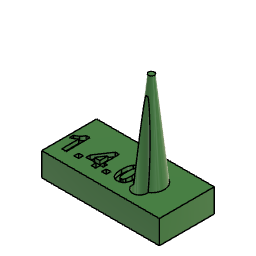
Straw_Thermocouple_Fastener_(STF)_V1.4.0 (Autodesk Fusion 360 design; units mm, degrees)
Autodesk Fusion 360 part; units mm, degrees
sketch "Sketch1" plane through (0, 0, 0) normal (0, 0, 1) x (1, 0, 0) in component "Component"
  circle A0 centre (0, 0) radius 1.625
  dimension "d1" = 3.25
  constraint coincident A0.centre origin
  measures "d1" diameter of A0
ref_plane "WorkPlane1" through (0, 0, 12) normal (0, 0, 1) x (1, 0, 0) in component "Component"
sketch "Sketch2" plane through (0, 0, 12) normal (0, 0, 1) x (1, 0, 0) in component "Component"
  circle A0 centre (0, 0) radius 0.375
  dimension "d3" = 0.75
  constraint coincident A0.centre origin
  measures "d3" diameter of A0
loft "Loft1" add profiles "Sketch1", "Sketch2" section 1 section 2 in component "Component"
sketch "Sketch3" plane through (0, 0, 0) normal (0, 0, -1) x (1, 0, 0) in component "Component"
  circle A0 centre (0, 0) radius 1.625
  line L0 (0, 0) -> (0.2762, 0)
  circle A1 centre (0, 1.5) radius 0.75
  line L1 (4.5, 3.5) -> (-10.5, 3.5)
  line L2 (-10.5, 3.5) -> (-10.5, -3.5)
  line L3 (-10.5, -3.5) -> (4.5, -3.5)
  line L4 (4.5, -3.5) -> (4.5, 3.5)
  line L5 (4.5, 3.5) -> (-10.5, -3.5) construction
  line L6 (-10.5, 3.5) -> (4.5, -3.5) construction
  point P0 (-3, 0)
  dimension "d6" = 1.5
  dimension "d25" = 15
  dimension "d26" = 7
  constraint coincident A0.centre L0.start
  constraint horizontal L0
  constraint horizontal L1
  constraint perpendicular L1 L2
  constraint parallel L1 L3
  constraint parallel L2 L4
  constraint coincident L5 P0
  constraint coincident L6 P0
  measures "d6" diameter of A1
  measures "d25" distance of L2.end L3.end
  measures "d26" distance of L1.end L2.end
extrude "Extrude2" add sketch "Sketch3" along normal blind 3.5 contours A0 A1 | L1 L2 L3 L4 picked at (0.0408, -0.8297) in component "Component"
sketch "Sketch4" plane through (0, 0, -3.5) normal (0, 0, -1) x (1, 0, 0) in component "Component"
  circle A0 centre (0, 1.5) radius 0.9262
  circle A1 centre (0, 1.5) radius 0.75
  line L0 (4.5, -3.5) -> (4.5, 3.5)
  line L1 (4.5, 3.5) -> (-10.5, 3.5)
  line L2 (-10.5, 3.5) -> (-10.5, -3.5)
  line L3 (-10.5, -3.5) -> (4.5, -3.5)
  constraint concentric A0 A1
extrude "Extrude4" cut sketch "Sketch4" against normal blind 13.3 contours A0 | A1 in component "Component"
extrude "Extrude6" cut 1 faces at (-7.295, -0.409, -3.5) along direction (0, 0, 1) blind 0.5 in component "Component"
sketch "Sketch1 (2)" plane through (0, 0, 0) normal (0, 0, 1) x (-1, 0, 0)
  arc A0 (0.913, 1.3442) -> (-0.913, 1.3442) centre (0, 1.5) ccw
  arc A1 (-0.913, 1.3442) -> (0.913, 1.3442) centre (0, 0) ccw
  line L0 (9.025, 1.5079) -> (2.5153, 1.4599) construction
  line L1 (2.5153, 1.4599) -> (2.5298, -0.5079) construction
  line L2 (2.5298, -0.5079) -> (9.0395, -0.4599) construction
  line L3 (9.0395, -0.4599) -> (9.025, 1.5079) construction
  line L4 (10.2238, -2.5) -> (10.2238, 3.5)
  line L5 (10.2238, 3.5) -> (10.2238, 0.5)
  line L6 (10.2238, 0.5) -> (-4.7762, 0.5)
  line L7 (-4.5, 3.5) -> (-4.5, -3.5)
  line L8 (-4.5, -3.5) -> (10.5, -3.5)
  line L9 (10.5, -3.5) -> (10.5, 3.5)
  line L10 (10.5, 3.5) -> (-4.5, 3.5)
  dimension "d22" = 3
  text T0 "1.4.0" font "Arial" height 3 bold align centre middle in box 6.5099 x 1.9678 at (9.025, 1.5079) x (-0.999973, -0.007371) y (0.007371, -0.999973) spacing 1 kerned
  constraint coincident L6
extrude "Extrude8" cut sketch "Sketch1 (2)" against normal blind 0.5 text T0 in component "Component"
component "Component" placed x (1, 0, 0) y (0, 1, 0) z (0, 0, 1) at (0, 0, 0)
